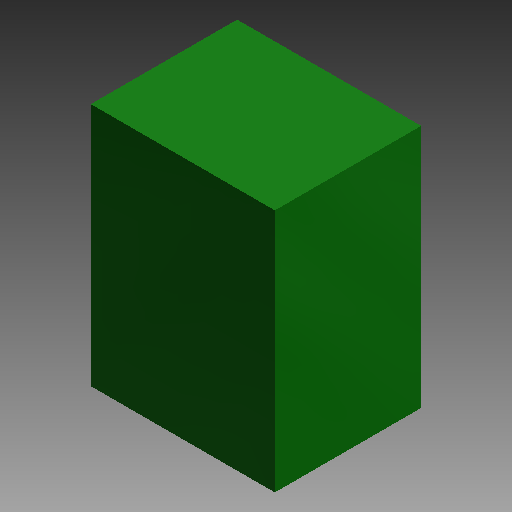
# Autodesk Inventor part: USB-B
Saved by Autodesk Inventor 2018.2 (Build 222227000, 227)
## iProperties
Part Number: USB-B
Material: Generic
Document SubType Name: Modeling
Designer: autocad
Appearance: PN61729, USB-B
Author: autocad
Autodesk Inventor part; units mm, degrees
ref_plane "YZ Plane" through (0, 0, 0) normal (1, 0, 0) x (0, 1, 0)
ref_plane "XZ Plane" through (0, 0, 0) normal (0, 1, 0) x (-1, 0, 0)
ref_plane "XY Plane" through (0, 0, 0) normal (0, 0, 1) x (1, 0, 0)
sketch "PN61729, USB-B_307" plane through (0, 0, 0) normal (0, 0, 1) x (1, 0, 0)
  line L0 (6.0452, 5.7404) -> (6.0452, -10.277)
  line L1 (6.0452, -10.277) -> (-6.027, -10.277)
  line L2 (-6.027, -10.277) -> (-6.027, 5.7404)
  line L3 (-6.027, 5.7404) -> (6.0452, 5.7404)
  constraints: 8 end point
extrude "Extrusion1" add sketch "PN61729, USB-B_307" along normal blind 9.6
body "Solid1"
